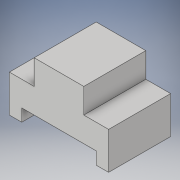
# Autodesk Inventor part: arthurWeiActivity 7.1#2
Saved by Autodesk Inventor 2018 (Build 220112000, 112)
## iProperties
Created: 2019-01-14
Part Number: arthurWeiActivity 7.1#2
Material: Generic
Document SubType Name: Modeling
Designer: This kid
Density: 1 g/cm^3
Appearance: Default
Author: This kid
Autodesk Inventor part; units mm, degrees
ref_plane "YZ Plane" through (0, 0, 0) normal (1, 0, 0) x (0, 1, 0)
ref_plane "XZ Plane" through (0, 0, 0) normal (0, 1, 0) x (-1, 0, 0)
ref_plane "XY Plane" through (0, 0, 0) normal (0, 0, 1) x (1, 0, 0)
sketch "Sketch1" plane through (0, 0, 0) normal (0, 0, 1) x (1, 0, 0)
  line L0 (-18.2066, -1.2573) -> (-11.8566, -1.2573)
  line L1 (-11.8566, -1.2573) -> (-11.8566, 5.0927)
  line L2 (-11.8566, 5.0927) -> (26.2434, 5.0927)
  line L3 (26.2434, 5.0927) -> (26.2434, -1.2573)
  line L4 (26.2434, -1.2573) -> (32.5934, -1.2573)
  line L5 (32.5934, -1.2573) -> (32.5934, 17.7927)
  line L6 (32.5934, 17.7927) -> (19.8934, 17.7927)
  line L7 (19.8934, 17.7927) -> (19.8934, 30.4927)
  line L8 (19.8934, 30.4927) -> (-5.5066, 30.4927)
  line L9 (-5.5066, 30.4927) -> (-5.5066, 17.7927)
  line L10 (-5.5066, 17.7927) -> (-18.2066, 17.7927)
  line L11 (-18.2066, 17.7927) -> (-18.2066, -1.2573)
  point P0 (0, 0)
  dimension "d0" = 6.35
  dimension "d1" = 6.35
  dimension "d2" = 38.1
  dimension "d3" = 6.35
  dimension "d4" = 19.05
  dimension "d5" = 12.7
  dimension "d6" = 12.7
  dimension "d7" = 25.4
  dimension "d8" = 12.7
  constraints: 24 end point, 7 perpendicular, 3 horizontal, 2 point on line
  measures "d0" distance of L0.start L0.end
  measures "d1" distance of L0.end L1.end
  measures "d2" distance of L1.end L2.end
  measures "d3" distance of L3.end L4.end
  measures "d4" distance of L4.end L5.end
  measures "d5" distance of L5.end L6.end
  measures "d6" distance of L6.end L7.end
  measures "d7" distance of L7.end L8.end
  measures "d8" distance of L9.end L10.end
extrude "Extrusion1" add sketch "Sketch1" along normal blind 31.75
body "Solid1"
